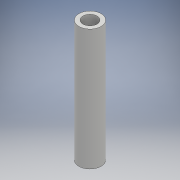
# Autodesk Inventor part: Separador de Base y Placa
Saved by Autodesk Inventor 2017 (Build 210142000, 142)
## iProperties
Part Number: Separador de Base y Placa
Material: Genérico
Document SubType Name: Modeling
Designer: fam
Density: 1 g/cm^3
Appearance: Valor por defecto
Author: fam
Autodesk Inventor part; units mm, degrees
ref_plane "YZ Plane" through (0, 0, 0) normal (1, 0, 0) x (0, 1, 0)
ref_plane "XZ Plane" through (0, 0, 0) normal (0, 1, 0) x (-1, 0, 0)
ref_plane "XY Plane" through (0, 0, 0) normal (0, 0, 1) x (1, 0, 0)
sketch "Boceto1" plane through (0, 0, 0) normal (0, 0, 1) x (1, 0, 0)
  circle A0 centre (0, 0) radius 1.75
  circle A1 centre (0, 0) radius 2.75
  dimension "d0" = 3.5
  dimension "d1" = 5.5
  constraints: 2 centre point, 1 coincident, 1 concentric
  measures "d0" diameter of A0
  measures "d1" diameter of A1
extrude "Extrusión1" add sketch "Boceto1" along normal blind 30
